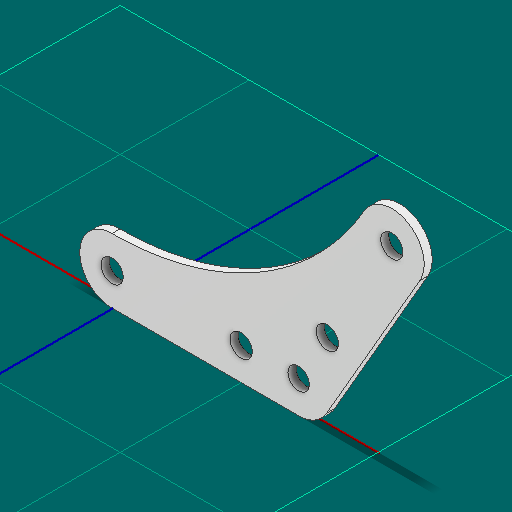
# Autodesk Inventor part: 60 Degree Gusset
Saved by Autodesk Inventor 2025 (Build 290162000, 162)
## iProperties
Created: 2024-10-22
Part Number: 60 Degree Gusset
Material: Acetal Resin, White
Document SubType Name: Modeling
Designer: averey
Density: 1.425 g/cm^3
Appearance: Smooth - White
Author: averey
Autodesk Inventor part; units mm, degrees
ref_plane "YZ Plane" through (0, 0, 0) normal (1, 0, 0) x (0, 1, 0)
ref_plane "XZ Plane" through (0, 0, 0) normal (0, 1, 0) x (-1, 0, 0)
ref_plane "XY Plane" through (0, 0, 0) normal (0, 0, 1) x (1, 0, 0)
sketch "main" plane through (0, 0, 0) normal (0, 0, 1) x (1, 0, 0)
  circle A0 centre (-6.1105, -12.0036) radius 2.1844
  circle A1 centre (-31.5105, -12.0036) radius 2.1844
  circle A2 centre (10.8754, -2.1968) radius 2.1844
  circle A3 centre (23.5754, 19.8003) radius 2.1844
  arc A4 (-31.5236, -5.6536) -> (-31.5105, -18.3536) centre (-31.5105, -12.0036) ccw
  arc A5 (29.0746, 16.6253) -> (18.0827, 22.9866) centre (23.5754, 19.8003) ccw
  arc A6 (-31.5236, -5.6536) -> (18.0827, 22.9866) centre (-31.6424, 51.8327) ccw
  line L0 (-31.5105, -18.3536) -> (5.2134, -18.3536)
  line L1 (29.0746, 16.6253) -> (10.7127, -15.1786)
  circle A7 centre (5.2134, -12.0036) radius 2.0955
  arc A8 (5.2134, -18.3536) -> (10.7127, -15.1786) centre (5.2134, -12.0036) ccw
  point P0 (-0.7926, -1.6009)
  dimension "d0" = 12.7
  dimension "d3" = 12.7
  dimension "d7" = 4.191
  dimension "d8" = 6.35
  measures "d0" diameter of A4
  measures "d3" diameter of A5
  measures "d7" diameter of A7
  measures "d8" radius of A8
sketch "Sketch1" plane through (0, 0, 0) normal (0, 0, 1) x (1, 0, 0)
  circle A0 centre (25.4, 0) radius 2.1844
  circle A1 centre (0, 0) radius 2.1844
  circle A2 centre (42.3858, 9.8068) radius 2.1844
  circle A3 centre (55.0858, 31.8038) radius 2.1844
  arc A4 (-0.0131, 6.35) -> (0, -6.35) centre (0, 0) ccw
  arc A5 (60.5851, 28.6288) -> (49.5932, 34.9902) centre (55.0858, 31.8038) ccw
  arc A6 (-0.0131, 6.35) -> (49.5932, 34.9902) centre (-0.132, 63.8362) ccw
  line L0 (0, -6.35) -> (36.7239, -6.35)
  line L1 (60.5851, 28.6288) -> (42.2232, -3.175)
  circle A7 centre (36.7239, 0) radius 2.0955
  arc A8 (36.7239, -6.35) -> (42.2232, -3.175) centre (36.7239, 0) ccw
  constraints: 1 other
extrude "Extrusion1" add sketch "Sketch1" along normal blind 1.5875
body "Solid1"
